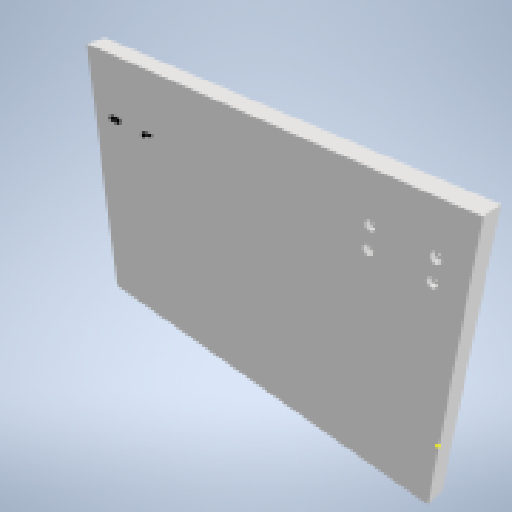
# Autodesk Inventor part: Base de mdf
Saved by Autodesk Inventor 2023 (Build 270158000, 158)
## iProperties
Created: 2022-09-27
Part Number: Base de mdf
Material: Generic
Document SubType Name: Modeling
Designer: kleber
Density: 1 g/cm^3
Appearance: Default
Author: kleber
Autodesk Inventor part; units mm, degrees
ref_plane "YZ Plane" through (0, 0, 0) normal (1, 0, 0) x (0, 1, 0)
ref_plane "XZ Plane" through (0, 0, 0) normal (0, 1, 0) x (-1, 0, 0)
ref_plane "XY Plane" through (0, 0, 0) normal (0, 0, 1) x (1, 0, 0)
sketch "Sketch1" plane through (0, 0, 0) normal (0, 0, 1) x (1, 0, 0)
  line L0 (-14.4097, -50.425) -> (-284.25, -50.425)
  line L1 (-284.25, 149.575) -> (-14.4097, 149.575)
  line L2 (0.6703, 149.575) -> (-299.3297, 149.575)
  line L3 (-299.3297, 149.575) -> (-299.3297, -50.425)
  line L4 (-299.3297, -50.425) -> (0.6703, -50.425)
  line L5 (0.6703, -50.425) -> (0.6703, 149.575)
  point P0 (0, 0)
  dimension "d4" = 200
  dimension "d30" = 300
  constraints: 12 end point, 3 parallel, 2 horizontal, 1 perpendicular
  measures "d4" distance of L0.end L1.start
  measures "d30" distance of L4.end L3.end
extrude "Extrusion1" add sketch "Sketch1" along normal blind 15
sketch "Sketch4" plane through (0, 0, 0) normal (0, 0, -1) x (-1, 0, 0)
  line L0 (299.3297, -50.425) -> (-0.6703, -50.425) projected
  line L1 (299.3297, 149.575) -> (299.3297, -50.425) projected
  line L2 (-0.6703, 149.575) -> (299.3297, 149.575) projected
  line L3 (-0.6703, -50.425) -> (-0.6703, 149.575) projected
  circle A0 centre (59.4097, 117.3225) radius 2.75
  circle A1 centre (59.4097, 102.3225) radius 2.75
  circle A2 centre (19.4097, 102.3225) radius 2.75
  circle A3 centre (19.4097, 117.3225) radius 2.75
  point P0 (0, 0)
  constraints: 4 centre point, 8 other
hole "Hole3" at (-19.4097, 117.3225, 0) at (-19.4097, 102.3225, 0) at (-59.4097, 102.3225, 0) at (-59.4097, 117.3225, 0) direction (0, 0, 1) diameter 3 end through all
sketch "Sketch5" plane through (0, 0, 15) normal (0, 0, 1) x (1, 0, 0)
  circle A0 centre (-19.4097, 117.3225) radius 3.5
  circle A1 centre (-19.4097, 102.3225) radius 3.5
  circle A2 centre (-59.4097, 102.3225) radius 3.5
  circle A3 centre (-59.4097, 117.3225) radius 3.5
  point P0 (0, 0)
  constraints: 4 centre point, 8 other
extrude "Extrusion2" cut sketch "Sketch5" against normal blind 4
sketch "Sketch6" plane through (0, 0, 15) normal (0, 0, 1) x (1, 0, 0)
  circle A0 centre (-276.75, 102.5725) radius 3.5
  circle A1 centre (-276.75, 114.5725) radius 3.5
  circle A2 centre (-241.75, 102.5725) radius 3.5
  circle A3 centre (-241.75, 114.5725) radius 3.5
  point P0 (0, 0)
  dimension "d54" = 7
  dimension "d55" = 7
  dimension "d56" = 7
  dimension "d57" = 7
  constraints: 4 centre point
  measures "d54" diameter of A0
  measures "d55" diameter of A1
  measures "d56" diameter of A2
  measures "d57" diameter of A3
extrude "Extrusion4" cut sketch "Sketch6" against normal blind 4
hole "Hole5" at (-276.75, 102.5725, 15) at (-276.75, 114.5725, 15) at (-241.75, 114.5725, 15) at (-241.75, 102.5725, 15) direction (0, 0, -1) diameter 3 end through all
body "Solid1"
